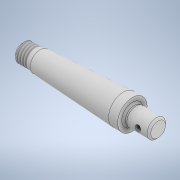
# Autodesk Inventor part: Рукоятка-8
Saved by Autodesk Inventor 2022 (Build 260153000, 153)
## iProperties
Created: 2021-12-03
Part Number: Рукоятка-8
Material: Типовые
Document SubType Name: Modeling
Designer: Украинцев
Density: 1 g/cm^3
Appearance: По умолчанию
Author: Украинцев
Autodesk Inventor part; units mm, degrees
ref_plane "YZ Plane" through (0, 0, 0) normal (1, 0, 0) x (0, 1, 0)
ref_plane "XZ Plane" through (0, 0, 0) normal (0, 1, 0) x (-1, 0, 0)
ref_plane "XY Plane" through (0, 0, 0) normal (0, 0, 1) x (1, 0, 0)
sketch "Эскиз1" plane through (0, 0, 0) normal (0, 1, 0) x (-1, 0, 0)
  line L0 (0, 0) -> (0, -5)
  line L1 (0, -5) -> (12, -5)
  line L2 (14, 0) -> (14, -4.75)
  line L3 (14, -4.75) -> (13, -4.75)
  line L4 (12, -4.75) -> (12, -5)
  line L5 (14, 0) -> (14, -8)
  line L6 (14, -8) -> (19, -8)
  line L7 (19, 0) -> (64, 0)
  line L8 (64, -5) -> (64, -5.5)
  line L9 (64, -5.5) -> (19, -8)
  line L10 (64, -5.5) -> (64, -5)
  line L11 (64, -5) -> (74, -5)
  line L12 (74, -5) -> (74, 0)
  line L13 (74, 0) -> (0, 0)
  line L14 (14, -4.75) -> (14, -5.75)
  line L15 (14, -5.75) -> (13, -5.75)
  arc A0 (14, -5.75) -> (13, -4.75) centre (13, -5.75) ccw
  line L16 (13, -4.75) -> (12, -5)
  dimension "d0" = 5
  dimension "d1" = 12
  dimension "d3" = 2
  dimension "d5" = 5
  dimension "d6" = 45
  dimension "d7" = 5.5
  dimension "d8" = 0.5
  dimension "d9" = 10
  dimension "d25" = 1
  constraints: 34 end point, 9 perpendicular, 2 point on circle, 2 point on line, 2 vertical, 1 centre point, 1 coincident, 1 horizontal
  measures "d0" distance of L0.start L0.end
  measures "d1" distance of L0.end L1.end
  measures "d3" distance of L2.end L4.start
  measures "d5" distance of L5.end L6.end
  measures "d6" distance of L7.start L7.end
  measures "d7" distance of L7.end L8.end
  measures "d8" distance of L8.start L8.end
  measures "d9" distance of L8.start L11.end
  measures "d25" distance of L14.end L2.end
revolve "Вращение1" add sketch "Эскиз1" angle 360 about axis through (-74, 0, 0) along (1, 0, 0)
thread "Резьба1" size "M10x1.5" class "6g" standard "ANSI Metric M Profile" length 7.5
sketch "Эскиз2" plane through (0, 0, 0) normal (0, 1, 0) x (-1, 0, 0)
  line L0 (14, 5.0083) -> (6, 5)
  line L1 (12, 5) -> (0, 5) projected
  line L2 (6, 5) -> (9.0413, -6.3501)
  line L3 (6, 5) -> (17.7505, 5) construction
  line L4 (9.0413, -6.3501) -> (10.4902, -5.9619)
  line L5 (10.4902, -5.9619) -> (6.6566, 8.345)
  line L6 (6.6566, 8.345) -> (5.2077, 7.9567)
  line L7 (5.2077, 7.9567) -> (9.0413, -6.3501)
  point P0 (0, 0)
  point P1 (7.5525, 5.0016)
  dimension "d13" = 8
  dimension "d14" = 75
  dimension "d15" = 1.5
  dimension "d16" = 1.5
  constraints: 14 end point, 2 perpendicular, 1 collinear, 1 equal length, 1 horizontal, 1 midpoint
  measures "d13" distance of L0.start L0.end
  measures "d14" angle of L2 L3
  measures "d15" distance of L2.end L4.end
  measures "d16" distance of L5.end L6.end
revolve "Вращение2" cut sketch "Эскиз2" angle 360 about axis through (-5.2077, 0, 7.9567) along (-0.2588, 0, -0.9659)
chamfer "Фаска1" distance 1 angle 45 1 edges at (0, 0, 5)
chamfer "Фаска2" distance 1.6 angle 45 1 edges at (-74, 0, 5)
